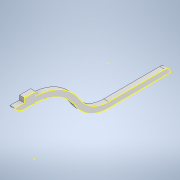
# Autodesk Inventor part: profile_dock
Saved by Autodesk Inventor 2020 (Build 240168000, 168)
## iProperties
Created: 2020-03-13
Part Number: profile_dock
Material: Generic
Document SubType Name: Modeling
Designer: erwin
Density: 1 g/cm^3
Appearance: Default
Author: erwin
Autodesk Inventor part; units mm, degrees
ref_plane "YZ Plane" through (0, 0, 0) normal (1, 0, 0) x (0, 1, 0)
ref_plane "XZ Plane" through (0, 0, 0) normal (0, 1, 0) x (-1, 0, 0)
ref_plane "XY Plane" through (0, 0, 0) normal (0, 0, 1) x (1, 0, 0)
sketch "Sketch1" plane through (0, 0, 0) normal (1, 0, 0) x (0, 1, 0)
  line L0 (12.0952, 0) -> (12.0952, 120)
  arc A0 (45.6451, 180.2938) -> (12.0952, 120) centre (83.0482, 120) ccw
  arc A1 (45.6451, 180.2938) -> (100.0539, 276) centre (-15.0339, 278.1084) ccw
  line L1 (88.0952, 300) -> (88.0952, 277.7802)
  arc A2 (40.548, 191.2386) -> (88.0952, 277.7802) centre (-15.0339, 278.1084) ccw
  arc A3 (40.548, 191.2386) -> (0.0952, 120) centre (83.0482, 120) ccw
  line L2 (0.0952, 120) -> (0.0952, 0)
  line L3 (100.0952, 300) -> (109, 300)
  line L4 (109, 300) -> (109, 276)
  line L5 (109, 276) -> (100, 276)
  arc A4 (100.0952, 320.3087) -> (88.0952, 300) centre (111.2804, 300) ccw
  line L6 (100.0952, 320.3087) -> (100.0952, 300)
  arc A5 (0.0952, -12) -> (12.0952, 0) centre (0.0952, 0) ccw
  line L7 (0.0952, -12) -> (0.0952, 0)
  line L8 (12.0952, 10) -> (0.0952, 10)
  line L9 (0.0952, 110) -> (12.0952, 110)
  point P0 (0, 0)
  point P1 (12.0952, 60)
  point P2 (0.0952, 0)
  dimension "d1" = 120
  dimension "d3" = 300
  dimension "d6" = 9
  dimension "d7" = 24
  dimension "d8" = 12
  dimension "d11" = 100
  dimension "d12" = 12
  constraints: 20 end point, 12 point on circle, 6 centre point, 5 point on line, 5 tangent, 2 horizontal, 2 parallel, 2 vertical, 1 collinear, 1 midpoint, 1 perpendicular
  measures "d1" distance of L0.start L0.end
  measures "d3" vertical distance of L0.start L3.start
  measures "d6" distance of L4.end L5.end
  measures "d7" distance of L3.end L4.end
  measures "d8" distance between parallel lines of L0 L2
  measures "d11" distance between parallel lines of L2 L6
  measures "d12" distance between parallel lines of L1 L6
extrude "Extrusion1" add sketch "Sketch1" along normal blind 10
sketch "Sketch2" plane through (10, 0, 0) normal (1, 0, 0) x (0, 0, -1)
  arc A0 (-191.2386, 40.548) -> (-120, 0.0952) centre (-120, 83.0482) ccw projected
  line L0 (-120, 0.0952) -> (12, 0.0952) projected
  arc A1 (12, 0.0952) -> (0, 12.0952) centre (0, 0.0952) ccw projected
  line L1 (0, 12.0952) -> (-120, 12.0952) projected
  arc A2 (-180.2938, 45.6451) -> (-120, 12.0952) centre (-120, 83.0482) ccw projected
  arc A3 (-180.2938, 45.6451) -> (-276, 100.0539) centre (-278.1084, -15.0339) ccw projected
  line L2 (-276, 100.0539) -> (-276, 109) projected
  line L3 (-276, 109) -> (-300, 109) projected
  line L4 (-300, 109) -> (-300, 100.0952) projected
  line L5 (-300, 100.0952) -> (-320.3087, 100.0952) projected
  arc A4 (-320.3087, 100.0952) -> (-300, 88.0952) centre (-300, 111.2804) ccw projected
  line L6 (-300, 88.0952) -> (-277.7802, 88.0952) projected
  arc A5 (-191.2386, 40.548) -> (-277.7802, 88.0952) centre (-278.1084, -15.0339) ccw projected
  point P0 (0, 0)
body "Solid1"
